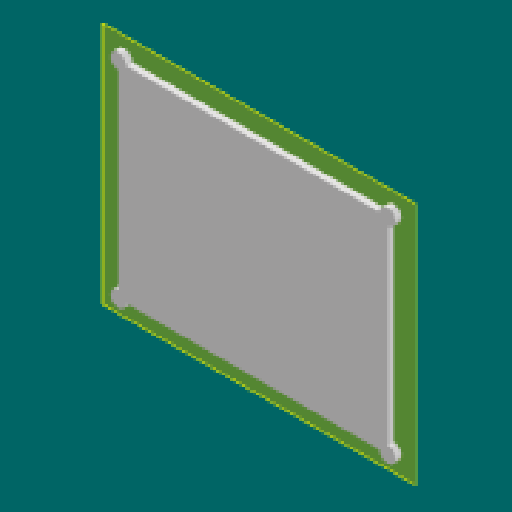
# Autodesk Inventor part: Part2
Saved by Autodesk Inventor 2025.2 (Build 292293000, 293)
## iProperties
Created: 2025-06-02
Part Number: Part2
Material: Generic
Document SubType Name: Modeling
Designer: ia088
Density: 1 g/cm^3
Appearance: Default
Author: ia088
Autodesk Inventor part; units mm, degrees
ref_plane "YZ Plane" through (0, 0, 0) normal (1, 0, 0) x (0, 1, 0)
ref_plane "XZ Plane" through (0, 0, 0) normal (0, 1, 0) x (-1, 0, 0)
ref_plane "XY Plane" through (0, 0, 0) normal (0, 0, 1) x (1, 0, 0)
ref_plane "Work Plane1" through (0, 0, 0) normal (0, 0, 1) x (1, 0, 0)
sketch "Sketch1" plane through (0, 0, 0) normal (0, 0, 1) x (1, 0, 0)
  arc A0 (-40, 32.5) -> (-42.5, 30) centre (-42.5, 32.5) ccw projected
  line L0 (-42.5, 30) -> (-42.5, -30) projected
  arc A1 (-42.5, -30) -> (-40, -32.5) centre (-42.5, -32.5) ccw projected
  line L1 (-40, -32.5) -> (40, -32.5) projected
  arc A2 (40, -32.5) -> (42.5, -30) centre (42.5, -32.5) ccw projected
  line L2 (42.5, -30) -> (42.5, 30) projected
  arc A3 (42.5, 30) -> (40, 32.5) centre (42.5, 32.5) ccw projected
  line L3 (40, 32.5) -> (-40, 32.5) projected
  arc A4 (-40.5, -28.5) -> (-38.5, -30.5) centre (-38.5, -28.5) ccw projected
  line L4 (-40.5, -28.5) -> (-40.5, 28.5) projected
  arc A5 (-38.5, 30.5) -> (-40.5, 28.5) centre (-38.5, 28.5) ccw projected
  line L5 (-38.5, 30.5) -> (38.5, 30.5) projected
  arc A6 (40.5, 28.5) -> (38.5, 30.5) centre (38.5, 28.5) ccw projected
  line L6 (40.5, 28.5) -> (40.5, -28.5) projected
  arc A7 (38.5, -30.5) -> (40.5, -28.5) centre (38.5, -28.5) ccw projected
  line L7 (38.5, -30.5) -> (-38.5, -30.5) projected
  circle A8 centre (-42.5, 32.5) radius 1.5 projected
  circle A9 centre (42.5, -32.5) radius 1.5 projected
  circle A10 centre (-42.5, -32.5) radius 1.5 projected
  circle A11 centre (42.5, 32.5) radius 1.5 projected
  point P0 (0, 0)
extrude "Extrusion1" add sketch "Sketch1" along normal blind 2 contours L3 A3 L2 A2 L1 A1 L0 A0 | L4 A5 L5 A6 L6 A7 L7 A4 | A8 | A9 | A10 | A11
sketch "Sketch2" plane through (0, 0, 0) normal (0, 0, -1) x (-1, 0, 0)
  circle A0 centre (42.5, 32.5) radius 1.5 projected
  circle A1 centre (-42.5, -32.5) radius 1.5 projected
  circle A2 centre (42.5, -32.5) radius 1.5 projected
  circle A3 centre (-42.5, 32.5) radius 1.5 projected
  arc A4 (42.5, 30) -> (40, 32.5) centre (42.5, 32.5) ccw projected
  line L0 (42.5, 30) -> (42.5, -30) projected
  arc A5 (40, -32.5) -> (42.5, -30) centre (42.5, -32.5) ccw projected
  line L1 (40, -32.5) -> (-40, -32.5) projected
  arc A6 (-42.5, -30) -> (-40, -32.5) centre (-42.5, -32.5) ccw projected
  line L2 (-42.5, -30) -> (-42.5, 30) projected
  arc A7 (-40, 32.5) -> (-42.5, 30) centre (-42.5, 32.5) ccw projected
  line L3 (-40, 32.5) -> (40, 32.5) projected
  arc A8 (38.5, -30.5) -> (40.5, -28.5) centre (38.5, -28.5) ccw projected
  line L4 (40.5, -28.5) -> (40.5, 28.5) projected
  arc A9 (40.5, 28.5) -> (38.5, 30.5) centre (38.5, 28.5) ccw projected
  line L5 (38.5, 30.5) -> (-38.5, 30.5) projected
  arc A10 (-38.5, 30.5) -> (-40.5, 28.5) centre (-38.5, 28.5) ccw projected
  line L6 (-40.5, 28.5) -> (-40.5, -28.5) projected
  arc A11 (-40.5, -28.5) -> (-38.5, -30.5) centre (-38.5, -28.5) ccw projected
  line L7 (-38.5, -30.5) -> (38.5, -30.5) projected
  line L8 (-42.5, -30) -> (-42.5, 30) projected
  circle A12 centre (-42.5, 32.5) radius 1.35
  circle A13 centre (-42.5, -32.5) radius 1.35
  circle A14 centre (42.5, 32.5) radius 1.35
  circle A15 centre (42.5, -32.5) radius 1.35
  point P0 (0, 0)
  dimension "d4" = 0.15
  dimension "d7" = 65
  dimension "d10" = 85
  constraints: 4 centre point, 1 horizontal, 1 vertical, 6 other
  measures "d4" radial gap between concentric circles of A3 A12
  measures "d7" distance of A3.centre A13.centre
  measures "d10" distance of A3.centre A14.centre
extrude "Extrusion2" add sketch "Sketch2" along normal blind 8.5 contours A12 | A13 | A14 | A15
body "Solid1"
